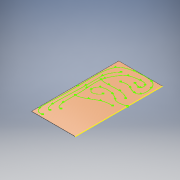
# Autodesk Inventor part: floor_50_100
Saved by Autodesk Inventor 2019 (Build 230136000, 136)
## iProperties
Created: 2020-04-28
Part Number: floor_50_100
Material: Wood (Birch)
Document SubType Name: Modeling
Designer: infinity
Density: 0.55 g/cm^3
Appearance: Birch - Natural Polished
Author: infinity
Autodesk Inventor part; units mm, degrees
ref_plane "YZ Plane" through (0, 0, 0) normal (1, 0, 0) x (0, 1, 0)
ref_plane "XZ Plane" through (0, 0, 0) normal (0, 1, 0) x (-1, 0, 0)
ref_plane "XY Plane" through (0, 0, 0) normal (0, 0, 1) x (1, 0, 0)
sketch "Sketch1" plane through (0, 0, 0) normal (0, 1, 0) x (-1, 0, 0)
  line L0 (0, 0) -> (15240, 0)
  line L1 (15240, 0) -> (15240, -30480)
  line L2 (15240, -30480) -> (0, -30480)
  line L3 (0, -30480) -> (0, 0)
  dimension "d0" = 30480
  dimension "d1" = 15240
  constraints: 8 end point, 2 parallel, 1 horizontal, 1 perpendicular
  measures "d0" distance of L0.end L1.end
  measures "d1" distance of L0.start L0.end
extrude "Extrusion1" add sketch "Sketch1" along normal blind 76.2
sketch "Sketch2" plane through (0, 76.2, 0) normal (0, 1, 0) x (1, 0, 0)
  spline S0 degree 4 poles (-12302.6973, 931.203) (-17173.3662, 219.5298) (-12488.7705, 8084.8735) (-17763.8572, 27977.3446) (-11067.1526, 30115.9847) (-3422.0832, 30805.6007) (-1140.1128, 28933.4401) (-484.8618, 22307.5949) (-4735.9773, 23376.5767) (-6031.0599, 25770.5448) (-8507.6327, 24434.7281) knots 0 0 0 0 0 0.30981 0.445334 0.558729 0.65371 0.738118 0.812118 1 1 1 1 1
  spline S1 degree 4 poles (-12302.6973, 3518.7471) (-16795.6726, 2413.0086) (-9996.8053, 23341.1053) (-16854.688, 21379.0887) (-11440.1826, 27453.5295) knots 0 0 0 0 0 1 1 1 1 1
  spline S2 degree 4 poles (-10836.4224, 5847.5367) (-13755.2218, 5346.2641) (-10862.9987, 15504.9268) (-15135.2644, 19296.3641) (-9847.8855, 28301.7276) (-6789.0431, 28154.0146) (-1934.6642, 29092.9084) (-3567.6287, 24348.1008) (-4003.6178, 26493.4636) (-5618.2086, 26504.7634) knots 0 0 0 0 0 0.350858 0.499555 0.627049 0.736202 0.819195 1 1 1 1 1
  spline S3 degree 3 poles (-12690.8289, 21767.8191) (-10028.0338, 20808.9853) (-5515.1302, 22800.5154) (-2599.4072, 20294.6577) knots 0 0 0 0 1 1 1 1
  line L0 (0, 0) -> (0, 30480) projected
  spline S4 degree 4 poles (0, 18267.7481) (-5328.9401, 16964.3909) (-1250.0418, 19610.3759) (-15654.4079, 22991.1059) (-11076.2708, 13708.9097) (-7990.1239, 17707.1136) knots 0 0 0 0 0 0.511471 1 1 1 1 1
  spline S5 degree 3 poles (-12432.0745, 12445.774) (-8513.0165, 13089.4506) (-7095.6008, 16351.3517) (-2599.4072, 15766.4556) knots 0 0 0 0 1 1 1 1
  point P0 (-14847.1156, 2440.6037)
  point P1 (-14847.1156, 15766.4556)
  point P2 (-13855.2237, 27884.7869)
  point P3 (-9456.3989, 30084.1993)
  point P4 (-3375.6705, 30041.0736)
  point P5 (-1348.7611, 27884.7869)
  point P6 (-1435.0126, 24348.4767)
  point P7 (-2944.4133, 23615.3392)
  point P8 (-5230.0771, 24434.7282)
  point P9 (-13855.2236, 5847.5367)
  point P10 (-13639.5949, 17362.1077)
  point P11 (-13639.5949, 23184.0818)
  point P12 (-12432.0745, 8219.4521)
  point P13 (-12690.8289, 16758.3474)
  point P14 (-12432.0745, 22795.9502)
  point P15 (-9111.393, 27582.9067)
  point P16 (-5618.2087, 28402.2957)
  point P17 (-3332.5449, 27755.4097)
  point P18 (-3332.5449, 26159.7575)
  point P19 (-3763.8022, 25901.0031)
  point P20 (-9844.5305, 21502.1782)
  point P21 (-6049.4659, 21588.4297)
  point P22 (-4324.4367, 18267.7481)
  point P23 (-6437.5974, 19475.2687)
  point P24 (-10577.6679, 19259.64)
  point P25 (-11440.1825, 17017.1019)
  point P26 (-9111.393, 13739.5461)
  point P27 (-6437.5975, 15240)
  constraints: 1 point on line, 41 other
body "Solid1"
